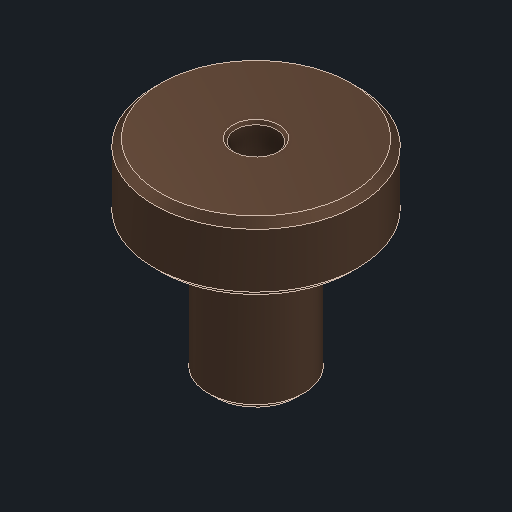
# Autodesk Inventor part: FM-306-10
Saved by Autodesk Inventor 2027.1 (Build 311270010, 270A)
## iProperties
Created: 2025-09-16
Part Number: FM-306-10
Material: Bronze, Soft Tin
Document SubType Name: Modeling
Designer: SD
Density: 8.874 g/cm^3
Appearance: Bronze - Satin
Mass: 10.1861 g
Surface Area: 8.99069 cm^2
Volume: 1.14786 cm^3
Project: Automatic Tea Steeping mechanism
Description: Flanged bronze bushing, 3×6×10 mm
Length: 15.000 mm
BOM-Mass: 0.01019
BOM-Area: 0.001
Diameter: 15.000 mm
Procurement: Fabricate - 1st round
Build Stage: 1
Preferred Material: Manufacturer Specification
Author: SD
Title: Bush
Autodesk Inventor part; units mm, degrees
ref_plane "YZ Plane" through (0, 0, 0) normal (1, 0, 0) x (0, 1, 0)
ref_plane "XZ Plane" through (0, 0, 0) normal (0, 1, 0) x (-1, 0, 0)
ref_plane "XY Plane" through (0, 0, 0) normal (0, 0, 1) x (1, 0, 0)
sketch "Sketch1" plane through (0, 0, 0) normal (0, 0, 1) x (1, 0, 0)
  line L0 (0, 0) -> (0, -15) construction
  line L1 (1.5, 0) -> (7.5, 0)
  line L2 (7.5, 0) -> (7.5, -5)
  line L3 (7.5, -5) -> (3.5, -5)
  line L4 (3.5, -5) -> (3.5, -15)
  line L5 (3.5, -15) -> (1.5, -15)
  line L6 (1.5, -15) -> (1.5, 0)
  dimension "d0" = 1.5
  dimension "d1" = 7.5
  dimension "d2" = 5
  dimension "d3" = 10
  dimension "Length" = 15
  dimension "d5" = 3.5
  constraints: 14 end point, 5 perpendicular, 1 horizontal, 1 horizontal alignment, 1 vertical
  measures "d0" distance between parallel lines of L0 L6
  measures "d1" distance between parallel lines of L0 L2
  measures "d2" distance of L1.end L2.end
  measures "d3" distance of L3.end L4.end
  measures "Length" distance of L0.start L0.end
  measures "d5" distance between parallel lines of L4 L0
revolve "Revolution1" add sketch "Sketch1" angle 360 about axis through (0, 0, 0) along (0, -1, 0)
chamfer "Chamfer1" distance 0.5 angle 45 3 edges at (-7.5, 0, 0) (-7.5, -5, 0) (-3.5, -15, 0)
chamfer "Chamfer2" distance 0.2 angle 45 2 edges at (-1.5, 0, 0) (-1.5, -15, 0)
equation "\"Diameter\" = 15"
body "Solid1"
